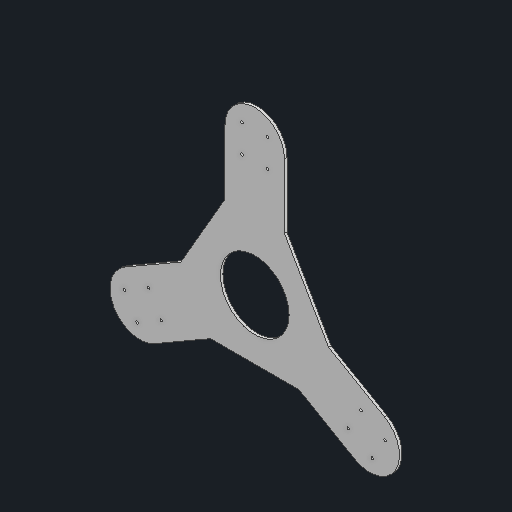
# Autodesk Inventor part: Bund
Saved by Autodesk Inventor 2026.1 (Build 301233020, 233B)
## iProperties
Created: 2025-11-07
Part Number: Bund
Material: Generic
Document SubType Name: Modeling
Designer: Mikke
Density: 1 g/cm^3
Appearance: Default
Author: Mikke
Autodesk Inventor part; units mm, degrees
ref_plane "YZ Plane" through (0, 0, 0) normal (1, 0, 0) x (0, 1, 0)
ref_plane "XZ Plane" through (0, 0, 0) normal (0, 1, 0) x (-1, 0, 0)
ref_plane "XY Plane" through (0, 0, 0) normal (0, 0, 1) x (1, 0, 0)
ref_plane "Work Plane1" through (0, 0, 0) normal (0, 0, 1) x (1, 0, 0)
sketch "Sketch1" plane through (0, 0, 0) normal (0, 0, 1) x (1, 0, 0)
  circle A0 centre (25, -136.9573) radius 110
  line L0 (-96.6901, -226.845) -> (-113.6901, -197.4001)
  line L1 (-101.8073, -229.7994) -> (-118.8073, -200.3545)
  line L2 (163.6901, -197.4001) -> (146.6901, -226.845)
  line L3 (168.8073, -200.3545) -> (151.8073, -229.7994)
  line L4 (8, 13.3733) -> (42, 13.3733)
  line L5 (8, 19.2822) -> (42, 19.2822)
  line L6 (25, -136.9573) -> (25, 19.2822)
  line L7 (25, -136.9573) -> (160.3073, -215.077)
  line L8 (25, -136.9573) -> (-110.3073, -215.077)
  line L9 (-10, -135.9724) -> (-10, 19.2822)
  line L10 (60, -135.9724) -> (60, 19.2822)
  line L11 (43.3529, -107.1388) -> (177.8073, -184.7661)
  line L12 (8.3529, -167.7605) -> (142.8073, -245.3879)
  line L13 (41.6471, -167.7605) -> (-92.8073, -245.3879)
  line L14 (6.6471, -107.1388) -> (-127.8073, -184.7661)
  arc A1 (142.8073, -245.3879) -> (177.8073, -184.7661) centre (160.3073, -215.077) ccw
  arc A2 (60, 19.2822) -> (-10, 19.2822) centre (25, 19.2822) ccw
  arc A3 (-127.8073, -184.7661) -> (-92.8073, -245.3879) centre (-110.3073, -215.077) ccw
  line L15 (25, -177.3718) -> (76.9615, -207.3718)
  line L16 (-10, -116.75) -> (-61.9615, -146.75)
  line L17 (-10, -116.75) -> (-10, -56.75)
  line L18 (60, -116.75) -> (60, -56.75)
  line L19 (60, -116.75) -> (111.9615, -146.75)
  line L20 (111.9615, -146.75) -> (60, -56.75)
  line L21 (-10, -56.75) -> (-61.9615, -146.75)
  line L22 (25, -177.3718) -> (-26.9615, -207.3718)
  line L23 (-26.9615, -207.3718) -> (76.9615, -207.3718)
  circle A4 centre (25, -136.9573) radius 40.4145
  point P0 (0, 0)
extrude "Extrusion1" add sketch "Sketch1" along normal blind 3 contours L10 A4 L6 A0 | A0 L9 A2 L10 | L11 A1 L12 A0 | A0 L7 A4 L11 | L6 A4 L9 A0 | L20 L11 L10 | A0 L12 A4 L7 | L14 A4 L8 A0 | A0 L13 A3 L14 | L9 L14 L21 | A0 L8 A4 L13 | L23 L13 L12
sketch "Sketch3" plane through (0, 0, 0) normal (0, 0, -1) x (-1, 0, 0)
  circle A0 centre (-40, -1.2646) radius 1.5 projected
  circle A1 centre (-10, -1.2646) radius 1.5 projected
  circle A2 centre (-10, 31.4848) radius 1.5 projected
  circle A3 centre (-40, 31.4848) radius 1.5 projected
  circle A4 centre (113.3751, -234.1687) radius 1.5 projected
  circle A5 centre (85.0133, -217.794) radius 1.5 projected
  circle A6 centre (100.0133, -191.8132) radius 1.5 projected
  circle A7 centre (128.3751, -208.1879) radius 1.5 projected
  circle A8 centre (-135.0133, -217.794) radius 1.5 projected
  circle A9 centre (-163.3751, -234.1687) radius 1.5 projected
  circle A10 centre (-178.3751, -208.1879) radius 1.5 projected
  circle A11 centre (-150.0133, -191.8132) radius 1.5 projected
  point P0 (0, 0)
extrude "Extrusion2" cut sketch "Sketch3" against normal blind 6
body "Solid1"
